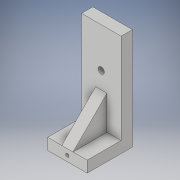
# Autodesk Inventor part: Verstrebung
Saved by Autodesk Inventor 2019 (Build 230136000, 136)
## iProperties
Created: 2021-06-13
Part Number: Verstrebung
Material: Generisch
Document SubType Name: Modeling
Designer: Bergi
Density: 1 g/cm^3
Appearance: Vorgabe
Author: Bergi
Autodesk Inventor part; units mm, degrees
ref_plane "YZ Plane" through (0, 0, 0) normal (1, 0, 0) x (0, 1, 0)
ref_plane "XZ Plane" through (0, 0, 0) normal (0, 1, 0) x (-1, 0, 0)
ref_plane "XY Plane" through (0, 0, 0) normal (0, 0, 1) x (1, 0, 0)
sketch "Skizze1" plane through (0, 0, 0) normal (0, 0, 1) x (1, 0, 0)
  line L0 (-17.5, -45) -> (17.5, -45)
  line L1 (17.5, -45) -> (17.5, 45)
  line L2 (17.5, 45) -> (-17.5, 45)
  line L3 (-17.5, 45) -> (-17.5, -45)
  line L4 (-17.5, -45) -> (17.5, 45) construction
  line L5 (17.5, -45) -> (-17.5, 45) construction
  point P0 (0, 0)
  dimension "d0" = 35
  dimension "d1" = 90
  constraints: 12 end point, 2 midpoint, 2 parallel, 1 horizontal, 1 perpendicular
  measures "d0" distance of L2.end L1.end
  measures "d1" distance of L1.end L0.end
extrude "Extrusion1" add sketch "Skizze1" along normal blind 10
sketch "Skizze2" plane through (0, 0, 10) normal (0, 0, 1) x (1, 0, 0)
  line L0 (-17.5, -45) -> (17.5, -45) projected
  line L1 (17.5, -45) -> (17.5, 45) projected
  line L2 (-17.5, -45) -> (17.5, -45)
  line L3 (17.5, -45) -> (17.5, -35)
  line L4 (17.5, -35) -> (-17.5, -35)
  line L5 (-17.5, -35) -> (-17.5, -45)
  point P0 (0, 0)
  dimension "d4" = 10
  constraints: 8 end point, 2 parallel, 1 horizontal, 1 perpendicular, 1 point on line
  measures "d4" distance of L3.end L2.end
extrude "Extrusion2" add sketch "Skizze2" along normal blind 30
sketch "Skizze3" plane through (0, 0, 0) normal (0, 0, -1) x (-1, 0, 0)
  line L0 (17.5, -45) -> (-17.5, -45) projected
  line L1 (-17.5, -45) -> (-17.5, -35) projected
  line L2 (-17.5, -35) -> (17.5, -35) projected
  line L3 (17.5, -35) -> (17.5, -45) projected
  line L4 (0, -63) -> (0, 63) projected
  line L5 (-17.5, -45) -> (-17.5, 45) projected
  line L6 (-17.5, -40) -> (17.5, -40)
  point P0 (0, 0)
  point P1 (0, 10)
  dimension "d7" = 50
  constraints: 2 end point, 2 point on line, 1 midpoint
  measures "d7" distance from line of point (0, 10) L6
hole "Bohrung1" at (0, 10, 0) direction (0, 0, 1) diameter 5.5 end through all counterbore diameter 10 counterbore depth 2.5
sketch "Skizze4" plane through (0, 0, 40) normal (0, 0, 1) x (1, 0, 0)
  line L0 (-17.5, -45) -> (17.5, -45) projected
  line L1 (17.5, -45) -> (17.5, -35) projected
  line L2 (17.5, -35) -> (-17.5, -35) projected
  line L3 (-17.5, -35) -> (-17.5, -45) projected
  line L4 (-17.5, -35) -> (17.5, -45) construction
  line L5 (-17.5, -35) -> (17.5, -35) construction
  line L6 (17.5, -35) -> (-17.5, -45) construction
  point P0 (0, 0)
  point P1 (0, -40)
  constraints: 4 end point, 1 midpoint
hole "Bohrung2" at (0, -40, 40) direction (0, 0, -1) diameter 2.9 end through all
sketch "Skizze5" plane through (0, 0, 0) normal (1, 0, 0) x (0, 1, 0)
  line L0 (7.25, 10) -> (12.75, 10) projected
  line L1 (7.25, 2.5) -> (12.75, 2.5) projected
  line L2 (45, 10) -> (-35, 10) projected
  line L3 (-35, 10) -> (-35, 40) projected
  line L4 (-35, 40) -> (-4.9612, 10)
  line L5 (10.0388, 10) -> (10.0388, -4.326) construction
  line L6 (-35, 40) -> (-35, 10)
  line L7 (-4.9612, 10) -> (-35, 10)
  point P0 (0, 0)
  dimension "d22" = 15
  constraints: 8 end point, 2 point on line, 1 collinear, 1 perpendicular, 1 vertical
  measures "d22" distance from line of L4.end L5
extrude "Extrusion3" add sketch "Skizze5" along normal mid plane 10
